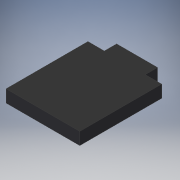
# Autodesk Inventor part: electromagnet_mnt_p2
Saved by Autodesk Inventor 2017 (Build 210142000, 142)
## iProperties
Created: 2018-03-20
Part Number: electromagnet_mnt_p2
Material: Generic
Document SubType Name: Modeling
Designer: Nic
Density: 1 g/cm^3
Appearance: Default
Author: Nic
Autodesk Inventor part; units mm, degrees
ref_plane "YZ Plane" through (0, 0, 0) normal (1, 0, 0) x (0, 1, 0)
ref_plane "XZ Plane" through (0, 0, 0) normal (0, 1, 0) x (-1, 0, 0)
ref_plane "XY Plane" through (0, 0, 0) normal (0, 0, 1) x (1, 0, 0)
sketch "Sketch1" plane through (0, 0, 0) normal (0, 0, 1) x (1, 0, 0)
  line L0 (9, 0) -> (9, -20)
  line L1 (9, -20) -> (-9, -20)
  line L2 (-9, -20) -> (-9, 0)
  line L3 (-5, 0) -> (-5, 3)
  line L4 (-5, 3) -> (5, 3)
  line L5 (5, 3) -> (5, 0)
  line L6 (-9, 0) -> (-5, 0)
  line L7 (5, 0) -> (9, 0)
  line L8 (0, 0) -> (0, 3) construction
  line L9 (0, 0) -> (-9, 0) construction
  dimension "d0" = 18
  dimension "d1" = 4
  dimension "d2" = 3
  dimension "d3" = 20
  constraints: 20 end point, 8 perpendicular, 3 horizontal, 3 parallel, 2 collinear, 1 midpoint, 2 other
  measures "d0" distance between parallel lines of L0 L2
  measures "d1" distance of L5.end L0.start
  measures "d2" distance of L3.start L3.end
  measures "d3" distance of L1.end L2.end
extrude "Extrusion1" add sketch "Sketch1" along normal blind 3
body "Solid1"
